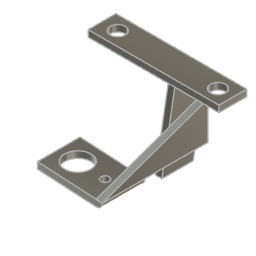
Mount v6 (Autodesk Fusion 360 design; units mm, degrees)
Autodesk Fusion 360 part; units mm, degrees
sketch "Sketch4" plane through (0, 0, 0) normal (0, 0, 1) x (1, 0, 0)
  line L0 (-47.7, 10.125) -> (47.7, 10.125)
  line L1 (47.7, 10.125) -> (47.7, -10.125)
  line L2 (47.7, -10.125) -> (-47.7, -10.125)
  line L3 (-47.7, -10.125) -> (-47.7, 10.125)
  line L4 (-47.7, 0) -> (47.7, 0) construction
  circle A0 centre (36.95, 0) radius 5.5
  line L5 (0.3455, 47) -> (0.3455, -29) construction
  circle A1 centre (-36.2591, 0) radius 5.5
  line L6 (42.45, 3.7083) -> (42.45, -3.7083) construction
  point P0 (47.7, 0)
  point P1 (-47.7, 0)
  point P2 (42.45, 0)
  dimension "d16" = 95.4
  dimension "d17" = 20.25
  dimension "d18" = 11
  dimension "d20" = 5.25
  constraint perpendicular L0 L1
  constraint perpendicular L2 L3
  constraint parallel L0 L2
  constraint midpoint L1 P0
  constraint midpoint L3 P1
  constraint coincident P1 L4.start
  constraint coincident P0 L4.end
  constraint midpoint L4 origin
  constraint coincident L4 A0.centre
  constraint vertical L5
  constraint symmetric A0 L5 A1
  constraint coincident L4 P2
  constraint coincident A0 P2
  constraint midpoint L6 P2
  constraint tangent A0 L6
  measures "d16" distance of L1 L3
  measures "d17" distance of L0.start L2.end
  measures "d18" diameter of A0
  measures "d20" distance of L1 L6
extrude "Extrude2" add sketch "Sketch4" along normal blind 4.7625
sketch "Sketch5" plane through (0, 0, 0) normal (0, 0, -1) x (1, 0, 0)
  circle A0 centre (36.95, 0) radius 5.5
  circle A1 centre (-36.2591, 0) radius 5.5
  line L0 (47.7, 10.125) -> (-47.7, 10.125)
  line L1 (-47.7, 10.125) -> (-47.7, -10.125)
  line L2 (-47.7, -10.125) -> (47.7, -10.125)
  line L3 (47.7, -10.125) -> (47.7, 10.125)
  line L4 (10.7, 15.5999) -> (15.4625, 15.5999)
  line L5 (15.4625, 15.5999) -> (15.4625, -14.8215)
  line L6 (10.7, -14.8215) -> (10.7, 15.5999)
  line L7 (10.7, -14.8215) -> (15.4625, -14.8215)
  dimension "d24" = 37
  dimension "d25" = 4.7625
  constraint horizontal L4
  constraint vertical L5
  constraint vertical L6
  constraint coincident L4.start L6.end
  constraint coincident L5.end L7.end
  constraint coincident L6.start L7.start
  constraint horizontal L7
  measures "d24" distance of L3 L6
  measures "d25" distance of L5 L6
extrude "Extrude3" add sketch "Sketch5" along normal blind 53.2375 contours L0 L2 L5 L6 | L0 L4 L5 L6 | L2 L5 L6 L7
sketch "Sketch6" plane through (15.4625, 0, 0) normal (1, 0, 0) x (0, 1, 0)
  line L0 (-10.125, 0) -> (-15.5999, 0)
  line L1 (-15.5999, 0) -> (-15.5999, -53.2375)
  line L2 (-15.5999, -53.2375) -> (14.8215, -53.2375)
  line L3 (14.8215, -53.2375) -> (14.8215, 0)
  line L4 (14.8215, 0) -> (10.125, 0)
  line L5 (10.125, 0) -> (-10.125, 0)
  line L6 (-10.125, 0) -> (10.125, 0)
  line L7 (10.125, 0) -> (10.125, -15)
  line L8 (-10.125, 0) -> (-19.5122, -53.2375)
  line L9 (10.125, -15) -> (3.3827, -53.2375)
  line L10 (-19.5122, -53.2375) -> (3.3827, -53.2375)
  point P0 (10.125, 0)
  dimension "d30" = 100
  constraint horizontal L6
  constraint vertical L7
  constraint coincident L0.start L5.end
  constraint coincident P0 L4.end
  constraint parallel L8 L9
  constraint coincident L7.end L9.start
  constraint horizontal L10
  constraint collinear L2 L10
  measures "d30" angle of L6 L8
extrude "Extrude4" cut sketch "Sketch6" against normal up to surface (4.7625 mm away) contours L0 L1 L8 | L2 L3 L4 L7 L9
extrude "Extrude5" add sketch "Sketch6" against normal up to surface (4.7625 mm away) contours L1 L8 L10
sketch "Sketch7" plane through (15.4625, 0, 0) normal (1, 0, 0) x (0, 1, 0)
  line L0 (3.3827, -53.2375) -> (10.125, -15)
  line L1 (10.125, -15) -> (10.125, 0)
  line L2 (10.125, 0) -> (-10.125, 0)
  line L3 (-10.125, 0) -> (-19.5122, -53.2375)
  line L4 (-19.5122, -53.2375) -> (3.3827, -53.2375)
  line L5 (-67.6425, -42.2375) -> (9.3575, -14.7375)
  line L6 (9.3575, -14.7375) -> (9.3575, -42.2375)
  line L7 (9.3575, -42.2375) -> (-67.6425, -42.2375)
  line L8 (-10.125, 4.7625) -> (10.125, 4.7625)
  dimension "d35" = 77
  dimension "d36" = 27.5
  dimension "d37" = 47
  constraint horizontal L7
  constraint perpendicular L6 L7
  measures "d35" distance of L5.start L6.end
  measures "d36" distance of L5.end L6.end
  measures "d37" distance of L7 L8
extrude "Extrude6" add sketch "Sketch7" along normal blind 4.7625 contours L0 L3 L5 L6 L7 | L0 L6 L7 | L3 L5 L7
sketch "Sketch8" plane through (0, 0, -42.2375) normal (0, 0, -1) x (1, 0, 0)
  line L0 (15.4625, -5.3223) -> (15.4625, -9.3575)
  line L1 (15.4625, -9.3575) -> (20.225, -9.3575)
  line L2 (20.225, -9.3575) -> (20.225, 67.6425)
  line L3 (20.225, 67.6425) -> (15.4625, 67.6425)
  line L4 (15.4625, 67.6425) -> (15.4625, 17.5726)
  line L5 (15.4625, 17.5726) -> (15.4625, -5.3223)
  line L6 (20.225, 67.6425) -> (-29.775, 65.0221)
  line L7 (-29.775, 65.0221) -> (-29.775, 34.0221)
  line L8 (-29.775, 34.0221) -> (20.225, 36.6425)
  line L9 (20.225, 36.6425) -> (20.225, 67.6425)
  circle A0 centre (-15.125, 50.2899) radius 9.65
  line L10 (-15.125, 40.6399) -> (-15.125, 59.9399) construction
  line L11 (-5.475, 50.2899) -> (-24.775, 50.2899) construction
  line L12 (-24.775, 58.5104) -> (-24.775, 42.0694) construction
  line L13 (-15.1316, 59.9399) -> (-15.1184, 59.9399) construction
  line L14 (-15.1316, 40.6399) -> (-15.1184, 40.6399) construction
  line L15 (-15.9351, 65.7475) -> (-14.3149, 34.8324) construction
  line L16 (15.4625, 51.8929) -> (-29.775, 49.5221) construction
  circle A1 centre (5.996, 51.3968) radius 3
  line L17 (-5.6407, 53.7042) -> (-5.3358, 47.8857) construction
  line L18 (2.8046, 54.9702) -> (3.1956, 47.5094) construction
  point P0 (-15.125, 50.2899)
  point P1 (-5.4882, 50.795)
  point P2 (3.0001, 51.2398)
  dimension "d40" = 3
  dimension "d41" = 50
  dimension "d42" = 31
  dimension "d44" = 19.3
  dimension "d45" = 5
  dimension "d47" = 30.9575
  dimension "d49" = 6
  dimension "d50" = 8.5
  constraint vertical L7
  constraint coincident L2.end L3.start
  constraint parallel L6 L8
  constraint parallel L2 L9
  constraint midpoint P0 L11
  constraint midpoint P0 L10
  constraint horizontal L11
  constraint vertical L10
  constraint coincident A0 L11.start
  constraint coincident A0 L10.start
  constraint midpoint L11.end L12
  constraint tangent A0 L12
  constraint midpoint L10.end L13
  constraint tangent A0 L13
  constraint symmetric L11 L13.start L14.start
  constraint symmetric L11 L13.end L14.end
  constraint perpendicular L6 L15
  constraint coincident L6 L15.start
  constraint coincident L8 L15.end
  constraint perpendicular L15 L16
  constraint coincident L7 L16.end
  constraint coincident L4 L16.start
  constraint midpoint L15 P0
  constraint coincident L16 P0
  constraint coincident P0 A0.centre
  constraint coincident L16 A1.centre
  constraint coincident A0 P1
  constraint coincident L16 P1
  constraint midpoint L17 P1
  constraint tangent A0 L17
  constraint coincident L16 P2
  constraint coincident A1 P2
  constraint midpoint L18 P2
  constraint tangent A1 L18
  measures "d40" angle of L3 L6
  measures "d41" distance of L7 L9
  measures "d42" distance of L6.end L7.end
  measures "d44" diameter of A0
  measures "d45" distance of L7 L12
  measures "d47" distance of L6 L8
  measures "d49" diameter of A1
  measures "d50" distance of L17 L18
extrude "Extrude7" add sketch "Sketch8" along normal blind 4.7625 contours L4 L6 L7 L8 | L2 L4 L6 L8 L9
fillet "Fillet1" radius 4.7625 1 edges at (20.225, -52.1425, -47)
equation "d21 = ( 3 / 16 ) * 1 in"
equation "d25 = ( 3 / 16 ) * 1 in"
equation "d26 = 58 mm - ( ( 3 / 16 ) * 1 in )"
equation "d30 = 90 deg + 10 deg"
equation "d38 = ( 3 / 16 ) * 1 in"
equation "d51 = ( 3 / 16 ) * 1 in"
equation "d54 = ( 3 / 16 ) * 1 in"
